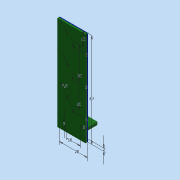
# Autodesk Inventor part: Led_Board_V1
Saved by Autodesk Inventor 2015 (Build 190159000, 159)
## iProperties
Created: 2014-12-24
Part Number: Led_Board_V1
Material: Generic
Document SubType Name: Modeling
Designer: Openlab
Density: 1 g/cm^3
Appearance: Smooth - Dark Forest Green
Author: Openlab
Autodesk Inventor part; units mm, degrees
ref_plane "YZ Plane" through (0, 0, 0) normal (1, 0, 0) x (0, 1, 0)
ref_plane "XZ Plane" through (0, 0, 0) normal (0, 1, 0) x (-1, 0, 0)
ref_plane "XY Plane" through (0, 0, 0) normal (0, 0, 1) x (1, 0, 0)
sketch "Sketch1" plane through (0, 0, 0) normal (0, 1, 0) x (-1, 0, 0)
  line L0 (20, 0) -> (0, 0)
  line L1 (0, 0) -> (0, -67)
  line L2 (0, -67) -> (20, -67)
  line L3 (20, -67) -> (20, 0)
  circle A0 centre (12.5, -10) radius 2.5
  circle A1 centre (12.5, -30) radius 2.5
  circle A2 centre (12.5, -50) radius 2.5
  line L4 (15, -63) -> (5, -63)
  line L5 (5, -63) -> (5, -65)
  line L6 (5, -65) -> (15, -65)
  line L7 (15, -65) -> (15, -63)
  dimension "d0" = 67
  dimension "d1" = 20
  dimension "d2" = 5
  dimension "d3" = 5
  dimension "d4" = 5
  dimension "d5" = 10
  dimension "d6" = 20
  dimension "d7" = 20
  dimension "d8" = 2
  dimension "d9" = 2
  dimension "d10" = 10
  dimension "d20" = 7.5
  dimension "d21" = 5
  constraints: 16 end point, 4 parallel, 3 centre point, 2 horizontal, 2 perpendicular, 2 vertical alignment, 1 coincident
  measures "d0" distance of L0.end L1.end
  measures "d1" distance of L1.end L2.end
  measures "d2" diameter of A0
  measures "d3" diameter of A1
  measures "d4" diameter of A2
  measures "d5" distance from line of L0 A0.centre
  measures "d6" distance of A1.centre A0.centre
  measures "d7" distance of A2.centre A1.centre
  measures "d8" distance between parallel lines of L2 L6
  measures "d9" distance of L6.end L4.start
  measures "d10" distance of L5.end L6.end
  measures "d20" distance from line of L3 A2.centre
  measures "d21" distance between parallel lines of L1 L5
extrude "Extrusion1" add sketch "Sketch1" against normal blind 1.5 contours L3 L2 L1 L0 | A0 | A1 | A2 | L7 L6 L5 L4
extrude "Extrusion2" add sketch "Sketch1" along normal blind 12 contours L7 L6 L5 L4
extrude "Extrusion3" add sketch "Sketch1" along normal blind 9 contours A0 | A1 | A2
fillet "Fillet1" radius 2 1 edges at (-10, 9, -10)
fillet "Fillet2" radius 2 1 edges at (-10, 9, -30)
fillet "Fillet3" radius 2 1 edges at (-10, 9, -50)
body "Solid1"
